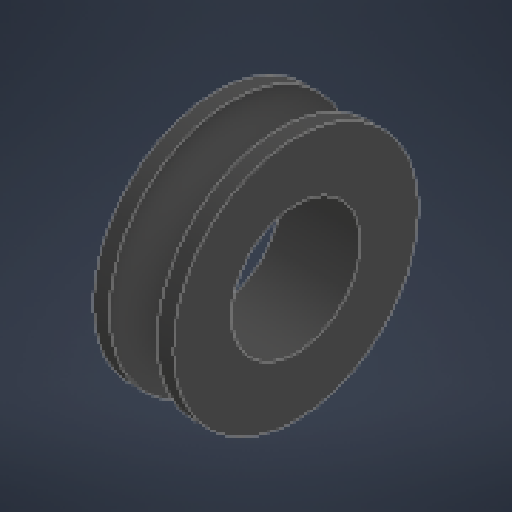
# Autodesk Inventor part: custombearing2
Saved by Autodesk Inventor 2026.1 (Build 301233020, 233B)
## iProperties
Created: 2025-12-15
Part Number: custombearing2
Material: 고무, 검은색
Document SubType Name: Modeling
Designer: jaewook
Density: 0.93 g/cm^3
Appearance: 고무 - 검은색
Author: jaewook
Autodesk Inventor part; units mm, degrees
ref_plane "YZ Plane" through (0, 0, 0) normal (1, 0, 0) x (0, 1, 0)
ref_plane "XZ Plane" through (0, 0, 0) normal (0, 1, 0) x (-1, 0, 0)
ref_plane "XY Plane" through (0, 0, 0) normal (0, 0, 1) x (1, 0, 0)
sketch "스케치1" plane through (0, 0, 0) normal (1, 0, 0) x (0, 1, 0)
  circle A0 centre (0, 0) radius 7.25
  circle A1 centre (0, 0) radius 8.3558
  dimension "d0" = 14.5
  constraints: 2 centre point, 1 coincident
  measures "d0" diameter of A0
extrude "돌출1" add sketch "스케치1" along normal mid plane 9
sketch "스케치2" plane through (0, 0, 0) normal (0, 0, 1) x (1, 0, 0)
  circle A0 centre (0, 12.1) radius 3.2
  circle A1 centre (0, 11.7) radius 2.8 construction
  line L0 (-4.5, 8.3558) -> (-4.5, -8.3558) projected
  line L1 (4.5, -8.3558) -> (4.5, 8.3558) projected
  line L2 (4.5, -8.3558) -> (4.5, 8.3558) projected
  line L3 (0, 0) -> (4.5, 0)
  line L4 (-4.5, 14.5) -> (4.5, 14.5)
  line L5 (-4.5, 8.3558) -> (-4.5, 14.5)
  line L6 (4.5, 8.3558) -> (4.5, 14.5)
  line L7 (-4.5, 13.8176) -> (4.5, 13.8176)
  line L8 (-4.5, 8.3558) -> (4.5, 8.3558)
  point P0 (2.6939, 14.1272)
  point P1 (-2.6939, 14.1272)
  point P2 (-2.7, 13.8176)
  point P3 (2.7, 13.8176)
  point P4 (-2.1166, 14.5)
  point P5 (2.1166, 14.5)
  point P6 (0.7101, 8.9798)
  point P7 (-0.7101, 8.9798)
  dimension "d3" = 6.4
  dimension "d4" = 5.6
  dimension "d6" = 29
  dimension "d8" = 5.4
  constraints: 12 end point, 4 point on line, 3 horizontal, 2 centre point, 2 perpendicular, 2 point on circle, 2 tangent, 2 vertical alignment, 1 midpoint, 1 parallel
  measures "d3" diameter of A0
  measures "d4" diameter of A1
  measures "d6" diameter of L4 L3
  measures "d8" distance of A0.end A0.start
revolve "회전1" add sketch "스케치2" angle 360 about axis through (0, 0, 0) along (1, 0, 0) contours A0 L7 L6 L8 L5
